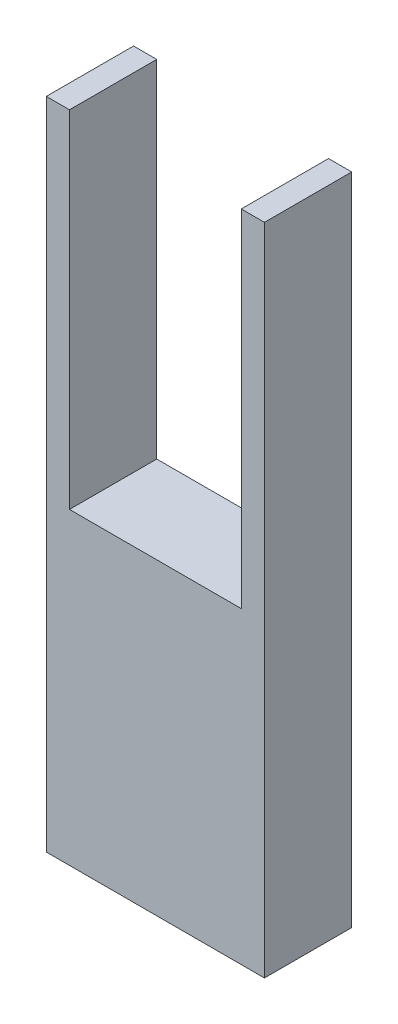
# Autodesk Inventor part: servoarm
Saved by Autodesk Inventor 2021.2 (Build 252289000, 289)
## iProperties
Created: 2021-03-03
Part Number: servoarm
Material: Generic
Document SubType Name: Modeling
Designer: zayda
Density: 1 g/cm^3
Appearance: Default
Author: zayda
Autodesk Inventor part; units mm, degrees
ref_plane "YZ Plane" through (0, 0, 0) normal (1, 0, 0) x (0, 1, 0)
ref_plane "XZ Plane" through (0, 0, 0) normal (0, 1, 0) x (-1, 0, 0)
ref_plane "XY Plane" through (0, 0, 0) normal (0, 0, 1) x (1, 0, 0)
sketch "Sketch1" plane through (0, 0, 0) normal (0, 0, 1) x (1, 0, 0)
  line L0 (0, 0) -> (25.4, 0)
  line L1 (25.4, 0) -> (25.4, 76.2)
  line L2 (25.4, 76.2) -> (0, 76.2)
  line L3 (0, 76.2) -> (0, 0)
  line L4 (12.7, 76.2) -> (22.606, 76.2)
  line L5 (12.7, 76.2) -> (2.794, 76.2)
  line L6 (12.7, 76.2) -> (2.7, 76.2)
  line L7 (12.7, 76.2) -> (22.7, 76.2)
  line L8 (2.7, 76.2) -> (22.7, 76.2)
  line L9 (22.7, 76.2) -> (22.7, 35.9)
  line L10 (22.7, 35.9) -> (2.7, 35.9)
  line L11 (2.7, 35.9) -> (2.7, 76.2)
  dimension "d0" = 25.4
  dimension "d1" = 76.2
  dimension "d14" = 10
  dimension "d15" = 10
  dimension "d16" = 20
  dimension "d17" = 40.3
  constraints: 24 end point, 4 perpendicular, 4 point on line, 2 horizontal, 2 parallel, 1 midpoint
  measures "d0" distance of L0.start L0.end
  measures "d1" distance of L0.end L1.end
  measures "d14" distance of L4.start L6.end
  measures "d15" distance of L4.start L7.end
  measures "d16" distance of L9.end L10.end
  measures "d17" distance of L8.end L9.end
extrude "Extrusion1" add sketch "Sketch1" along normal blind 10.16 contours L3 L2 L11 L10 L9 L1 L0
body "Solid1"
